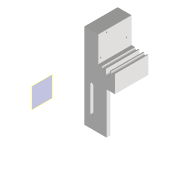
# Autodesk Inventor part: TIRFImager_Laserbase_v1
Saved by Autodesk Inventor 2022 (Build 260153000, 153)
## iProperties
Created: 2022-05-21
Part Number: TIRFImager_Laserbase_v1
Material: Generisch
Document SubType Name: Modeling
Designer: diederichbenedict
Density: 1 g/cm^3
Appearance: Vorgabe
Author: diederichbenedict
Autodesk Inventor part; units mm, degrees
ref_plane "YZ Plane" through (0, 0, 0) normal (1, 0, 0) x (0, 1, 0)
ref_plane "XZ Plane" through (0, 0, 0) normal (0, 1, 0) x (-1, 0, 0)
ref_plane "XY Plane" through (0, 0, 0) normal (0, 0, 1) x (1, 0, 0)
ref_plane "Arbeitsebene1" through (49.1253, 22.3022, -77.9087) normal (-1, 0, 0) x (0, -1, 0)
sketch "Skizze1" plane through (49.1253, 22.3022, -77.9087) normal (-1, 0, 0) x (0, -1, 0)
  line L0 (2.603, 4) -> (2.603, 19.5) construction
  line L1 (2.603, 19.5) -> (-10.897, 19.5) construction
  line L2 (-10.897, 19.5) -> (-10.897, 4) construction
  line L3 (-10.897, 4) -> (2.603, 4) construction
  circle A0 centre (6.603, 29.5) radius 1 construction
  circle A1 centre (-13.897, 23) radius 1 construction
  circle A2 centre (1.603, 1.5) radius 1 construction
  arc A3 (8.303, 27.8555) -> (9.303, 28.8555) centre (8.303, 28.8555) ccw construction
  line L4 (8.303, 27.8555) -> (5.5653, 27.8555) construction
  arc A4 (5.5653, 27.8555) -> (4.5653, 26.8555) centre (5.5653, 26.8555) ccw construction
  line L5 (4.5653, 26.8555) -> (4.5653, 0) construction
  arc A5 (3.5653, -1) -> (4.5653, 0) centre (3.5653, 0) ccw construction
  line L6 (3.5653, -1) -> (1, -1) construction
  arc A6 (0, 0) -> (1, -1) centre (1, 0) ccw construction
  line L7 (0, 0) -> (0, 1) construction
  arc A7 (0, 1) -> (-1, 2) centre (-1, 1) ccw construction
  line L8 (-1, 2) -> (-12.5347, 2) construction
  line L9 (-12.5347, 2) -> (-12.5347, 20.4723) construction
  arc A8 (-12.5347, 20.4723) -> (-13.5347, 21.4723) centre (-13.5347, 20.4723) ccw construction
  line L10 (-13.5347, 21.4723) -> (-15.397, 21.4723) construction
  arc A9 (-16.397, 22.4723) -> (-15.397, 21.4723) centre (-15.397, 22.4723) ccw construction
  line L11 (-16.397, 22.4723) -> (-16.397, 32) construction
  line L12 (-16.397, 32) -> (9.303, 32) construction
  line L13 (9.303, 32) -> (9.303, 28.8555) construction
  line L14 (-10.897, 4) -> (2.603, 4)
  line L15 (2.603, 4) -> (2.603, 26)
  line L16 (2.603, 26) -> (-10.897, 26)
  line L17 (-10.897, 26) -> (-10.897, 4)
  circle A10 centre (1.603, 1.5) radius 0.75
  circle A11 centre (6.603, 29.5) radius 0.75
  circle A12 centre (-13.897, 23) radius 0.75
  line L18 (71.478, -4) -> (23.478, -4) projected
  line L19 (71.478, 28) -> (23.478, 28) projected
  line L20 (-16.397, -4) -> (13.603, -4)
  line L21 (13.603, -4) -> (13.603, 32)
  line L22 (13.603, 32) -> (-16.397, 32)
  line L23 (-16.397, 32) -> (-16.397, -4)
  point P0 (22.3022, 77.9087)
  dimension "d0" = 22
  dimension "d1" = 1.5
  dimension "d2" = 1.5
  dimension "d3" = 1.5
  dimension "d4" = 30
  constraints: 16 end point, 4 parallel, 3 centre point, 3 coincident, 2 horizontal, 2 perpendicular
  measures "d0" distance of L15.end L14.end
  measures "d1" diameter of A10
  measures "d2" diameter of A11
  measures "d3" diameter of A12
  measures "d4" distance of L22.end L21.end
extrude "Extrusion1" add sketch "Skizze1" against normal blind 15
sketch "Skizze2" plane through (49.1253, 8.6992, -81.9087) normal (0, 0, -1) x (-1, 0, 0)
  line L0 (0, 0) -> (-15, 0) projected
  line L1 (0, -9.875) -> (0, 0)
  line L2 (0, 0) -> (-15, 0)
  line L3 (0, 0) -> (-31, 0)
  line L4 (-31, 0) -> (-31, -17)
  line L5 (-31, -17) -> (0, -17)
  line L6 (0, -17) -> (0, 0)
  line L7 (-15, 0) -> (-33, 0)
  line L8 (-33, 0) -> (-33, 2)
  line L9 (-33, 2) -> (-15, 2)
  line L10 (-15, 2) -> (-15, 0)
  line L11 (-33, 0) -> (-31, 0)
  line L12 (-31, 0) -> (-31, -17)
  line L13 (-31, -17) -> (-33, -17)
  line L14 (-33, -17) -> (-33, 0)
  point P0 (49.1253, -8.6992)
  dimension "d7" = 18
  dimension "d8" = 2
  dimension "d16" = 17
  constraints: 28 end point, 6 parallel, 4 perpendicular, 3 horizontal, 1 vertical
  measures "d7" distance of L8.end L9.end
  measures "d8" distance of L7.end L8.end
  measures "d16" distance between parallel lines of L0 L5
extrude "Extrusion2" add sketch "Skizze2" against normal up to surface (36 mm away)
sketch "Skizze3" plane through (64.1253, 38.6992, -81.9087) normal (0, 0, -1) x (-1, 0, 0)
  circle A0 centre (-10.4161, -44.1145) radius 1.635 projected
  line L0 (6.5932, -35.385) -> (6.5932, -27.885) projected
  line L1 (6.5932, -27.885) -> (-3.9542, -27.885) projected
  arc A1 (-7.1258, -27.885) -> (-3.9542, -27.885) centre (-5.54, -28.625) ccw projected
  line L2 (-7.1258, -27.885) -> (-8.35, -27.885) projected
  line L3 (-8.35, -27.885) -> (-8.35, -32.375) projected
  arc A2 (-12.55, -32.375) -> (-8.35, -32.375) centre (-10.45, -32.375) ccw projected
  line L4 (-12.55, -32.375) -> (-12.55, -27.885) projected
  line L5 (-12.55, -27.885) -> (-13.7742, -27.885) projected
  arc A3 (-16.9458, -27.885) -> (-13.7742, -27.885) centre (-15.36, -28.625) ccw projected
  line L6 (-16.9458, -27.885) -> (-21.2399, -27.885) projected
  line L7 (-21.2399, -27.885) -> (-21.2399, -62.885) projected
  line L8 (-21.2399, -62.885) -> (-20.9068, -62.885) projected
  line L9 (-20.9068, -62.885) -> (6.5932, -35.385) projected
  circle A4 centre (-5.54, -28.625) radius 1.75
  circle A5 centre (-10.45, -32.375) radius 2.1
  circle A6 centre (-15.36, -28.625) radius 1.75
  line L10 (-8.35, -32.375) -> (-12.55, -32.375)
  line L11 (-12.55, -32.375) -> (-12.55, -26.875)
  line L12 (-12.55, -26.875) -> (-8.35, -26.875)
  line L13 (-8.35, -26.875) -> (-8.35, -32.375)
  point P0 (64.1253, -38.6992)
  point P1 (-13.7742, -27.885)
  point P2 (-16.9458, -27.885)
  point P3 (-12.55, -27.885)
  point P4 (-8.35, -27.885)
  point P5 (-3.9542, -27.885)
  point P6 (-7.1258, -27.885)
  constraints: 8 end point, 3 coincident, 2 centre point, 2 concentric, 2 parallel, 1 horizontal, 1 horizontal alignment, 1 perpendicular, 3 other
extrude "Extrusion3" cut sketch "Skizze3" against normal through all contours A1 A4 | L3 A5 L4 L11 L12 L13 | A6 A3 | L10 A5 | A2 L10
sketch "Skizze4" plane through (49.1253, 38.6992, -45.9087) normal (0, 0, 1) x (1, 0, 0)
  line L0 (24, -92.2118) -> (24, -44.2118) projected
  line L1 (35, -39.875) -> (0, -39.875) projected
  line L2 (0, -39.875) -> (24, -39.875)
  line L3 (24, -39.875) -> (24, -92.2118)
  line L4 (24, -92.2118) -> (0, -92.2118)
  line L5 (0, -92.2118) -> (0, -39.875)
  circle A0 centre (8, -87.2118) radius 1.4 projected
  circle A1 centre (8, -49.2118) radius 1.4 projected
  line L6 (8, -78.1916) -> (8, -50.418) construction
  line L7 (9.5, -78.1916) -> (9.5, -50.418)
  line L8 (6.5, -50.418) -> (6.5, -78.1916)
  arc A2 (6.5, -78.1916) -> (9.5, -78.1916) centre (8, -78.1916) ccw
  arc A3 (9.5, -50.418) -> (6.5, -50.418) centre (8, -50.418) ccw
  point P0 (-49.1253, -38.6992)
  point P1 (8, -64.3048)
  point P2 (24, -44.2118)
  dimension "d13" = 3
  constraints: 16 end point, 4 point on circle, 4 tangent, 3 parallel, 2 centre point, 1 horizontal, 1 midpoint, 1 perpendicular, 1 vertical, 1 other
  measures "d13" diameter of A3
ref_plane "Arbeitsebene2" through (41.1253, -49.1758, -49.9087) normal (0, 0, 1) x (1, 0, 0)
extrude "Extrusion4" add sketch "Skizze4" against normal up to surface (4 mm away) contours L4 L5 L1 L3 L0 | A0 | A1 A3 picked at (8.0343, -48.5576)
sketch "Skizze5" plane through (64.1253, 38.6992, -81.9087) normal (0, 0, -1) x (-1, 0, 0)
  circle A0 centre (-10.4161, -44.1145) radius 1.635 projected
  point P0 (64.1253, -38.6992)
extrude "Extrusion5" cut sketch "Skizze5" against normal blind 10
sketch "Skizze6" plane through (49.1253, -8.3008, -81.9087) normal (0, -1, 0) x (1, 0, 0)
  circle A0 centre (8, 16) radius 2.5 projected
  circle A1 centre (8, 16) radius 4
  point P0 (-49.1253, 81.9087)
  dimension "d19" = 8
  constraints: 1 centre point, 1 coincident
  measures "d19" diameter of A1
extrude "Extrusion6" cut sketch "Skizze6" against normal blind 37 contours A0 | A1
sketch "Skizze7" plane through (49.1253, 38.6992, -45.9087) normal (0, 0, 1) x (1, 0, 0)
  line L0 (4, -19) -> (12, -19) projected
  line L1 (0.1, -13) -> (-7.6, -13)
  line L2 (-7.6, -13) -> (8, -13)
  line L3 (8, -13) -> (8, -19)
  line L4 (0, -5) -> (15, -20)
  line L5 (0, -5) -> (21.2132, -5) construction
  line L6 (15, 0) -> (15, -28) projected
  line L7 (0, 0) -> (0, -25.7) projected
  line L8 (0, -5.5) -> (15, -5.5) projected
  line L9 (15, -5.5) -> (15, -19) projected
  line L10 (0.5, -5.5) -> (15, -5.5)
  line L11 (15, -20) -> (15, -5.5)
  line L12 (1.9966, -5.5) -> (15, -18.5034)
  point P0 (-49.1253, -38.6992)
  dimension "d22" = 45
  dimension "d23" = 1.0582
  constraints: 16 end point, 7 point on line, 4 horizontal, 1 collinear, 1 equal length, 1 midpoint, 1 perpendicular, 2 other
  measures "d22" angle of L4 L5
  measures "d23" distance between parallel lines of L12 L4
extrude "Extrusion7" add sketch "Skizze7" against normal up to surface (28 mm away) contours L4 L8 L12 L6 | L8 L6 L12
